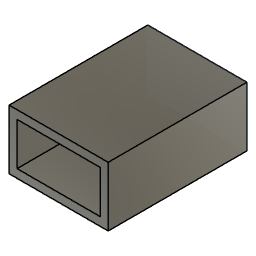
Panasonic DP-UB450 Remote Wall Mount (Autodesk Fusion 360 design; units mm, degrees)
Autodesk Fusion 360 part; units mm, degrees
sketch "Sketch1" plane through (0, 0, 0) normal (0, 0, 1) x (1, 0, 0)
  line L0 (25, -35) -> (-25, -35)
  line L1 (-25, -35) -> (-25, 35)
  line L2 (-25, 35) -> (25, 35)
  line L3 (25, 35) -> (25, -35)
  line L4 (25, -35) -> (-25, 35) construction
  line L5 (-25, -35) -> (25, 35) construction
  dimension "d1" = 50
  dimension "d2" = 70
  constraint horizontal L0
  constraint perpendicular L0 L1
  constraint parallel L0 L2
  constraint parallel L1 L3
  constraint coincident L4 origin
  constraint coincident L5 origin
  measures "d1" distance of L1 L3
  measures "d2" distance of L0 L2
extrude "Extrude1" add sketch "Sketch1" along normal blind 30
sketch "Sketch2" plane through (0, 35, 0) normal (0, 1, 0) x (-1, 0, 0)
  line L0 (-25, 0) -> (25, 0)
  line L1 (25, 0) -> (25, 30)
  line L2 (25, 30) -> (-25, 30)
  line L3 (-25, 30) -> (-25, 0)
sketch "Sketch3" plane through (0, -35, 0) normal (0, -1, 0) x (1, 0, 0)
  line L0 (-25, 0) -> (25, 0)
  line L1 (25, 0) -> (25, 30)
  line L2 (25, 30) -> (-25, 30)
  line L3 (-25, 30) -> (-25, 0)
  line L4 (-20.9844, 25.7659) -> (21.0156, 25.7659)
  line L5 (21.0156, 25.7659) -> (21.0156, 4.2659)
  line L6 (21.0156, 4.2659) -> (-20.9844, 4.2659)
  line L7 (-20.9844, 4.2659) -> (-20.9844, 25.7659)
  dimension "d5" = 42
  dimension "d6" = 21.5
  constraint horizontal L4
  constraint vertical L5
  constraint horizontal L6
  constraint vertical L7
  measures "d5" distance of L5 L7
  measures "d6" distance of L4 L6
extrude "Extrude2" cut sketch "Sketch3" against normal blind 65 contours L4 L5 L6 L7
